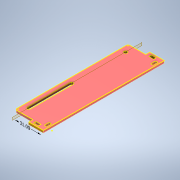
# Autodesk Inventor part: chassis_1_2
Saved by Autodesk Inventor 2022 (Build 260153000, 153)
## iProperties
Created: 2023-03-24
Part Number: chassis_1_2
Material: 一般
Document SubType Name: Modeling
Designer: Johnny Jou
Density: 79.16 g/cm^3
Appearance: 熔接 - 黃銅
Mass: 1010.18 g
Surface Area: 100.717 cm^2
Volume: 12.7613 cm^3
Author: Johnny Jou
Autodesk Inventor part; units mm, degrees
ref_plane "YZ Plane" through (0, 0, 0) normal (1, 0, 0) x (0, 1, 0)
ref_plane "XZ Plane" through (0, 0, 0) normal (0, 1, 0) x (-1, 0, 0)
ref_plane "XY Plane" through (0, 0, 0) normal (0, 0, 1) x (1, 0, 0)
sketch "草圖1" plane through (0, 0, 0) normal (0, 1, 0) x (-1, 0, 0)
  line L0 (0, 0) -> (0, -140)
  line L1 (15, -140) -> (15, 0)
  line L2 (6, 0) -> (6, 3)
  line L3 (6, 3) -> (14.1, 3)
  line L4 (14.1, 3) -> (14.1, 0)
  line L5 (15, 0) -> (14.1, 0)
  line L6 (6, 0) -> (0, 0)
  line L7 (6, -140) -> (6, -143)
  line L8 (6, -143) -> (14.1, -143)
  line L9 (14.1, -143) -> (14.1, -140)
  line L10 (0, -140) -> (6, -140)
  line L11 (14.1, -140) -> (15, -140)
  dimension "d1" = 15
  dimension "d2" = 3
  dimension "d3" = 8.1
  dimension "d4" = 6
  dimension "d5" = 3
  dimension "d6" = 140
  dimension "d7" = 6
  dimension "d8" = 8.1
  dimension "d9" = 15
  dimension "d10" = 140
  constraints: 24 end point, 7 parallel, 4 horizontal, 2 perpendicular, 1 coincident
  measures "d1" distance of L1.end L0.start
  measures "d2" distance of L3.end L4.end
  measures "d3" distance of L2.end L3.end
  measures "d4" distance between parallel lines of L0 L2
  measures "d5" distance of L8.end L9.end
  measures "d6" distance of L0.start L0.end
  measures "d7" distance between parallel lines of L0 L7
  measures "d8" distance of L7.end L8.end
  measures "d9" distance between parallel lines of L0 L1
  measures "d10" distance of L1.start L1.end
extrude "擠出1" add sketch "草圖1" along normal blind 3
sketch "草圖2" plane through (0, 3, 0) normal (0, 1, 0) x (1, 0, 0)
  line L0 (-11, 1) -> (-8, 1)
  line L1 (-8, 1) -> (-8, 7)
  line L2 (-8, 7) -> (-11, 7)
  line L3 (-11, 7) -> (-11, 1)
  line L4 (0, 0) -> (0, 140) projected
  line L5 (-6, 0) -> (0, 0) projected
  line L6 (-11, 133) -> (-8, 133)
  line L7 (-8, 133) -> (-8, 139)
  line L8 (-8, 139) -> (-11, 139)
  line L9 (-11, 139) -> (-11, 133)
  line L10 (0, 140) -> (-6, 140) projected
  line L11 (-15, 140) -> (-15, 0) projected
  dimension "d13" = 6
  dimension "d14" = 3
  dimension "d16" = 1
  dimension "d17" = 6
  dimension "d18" = 3
  dimension "d20" = 1
  dimension "d33" = 4
  dimension "d34" = 4
  constraints: 16 end point, 4 parallel, 2 horizontal, 2 perpendicular
  measures "d13" distance of L2.end L0.start
  measures "d14" distance of L1.end L2.end
  measures "d16" distance between parallel lines of L5 L0
  measures "d17" distance of L8.end L6.start
  measures "d18" distance of L6.start L6.end
  measures "d20" distance between parallel lines of L10 L8
  measures "d33" distance between parallel lines of L11 L3
  measures "d34" distance between parallel lines of L11 L9
extrude "擠出2" cut sketch "草圖2" against normal up to surface (3 mm away)
sketch "草圖4" plane through (0, 3, 0) normal (0, 1, 0) x (1, 0, 0)
  line L0 (-44, 0) -> (-15, 0)
  line L1 (-15, 0) -> (-15, 140)
  line L2 (-15, 140) -> (-44, 140)
  line L3 (-46, 138) -> (-46, 2)
  line L4 (-15, 140) -> (-15, 0) projected
  line L5 (0, 140) -> (-6, 140) projected
  line L6 (-6, 0) -> (0, 0) projected
  line L7 (-39, 10) -> (-39, 63) construction
  line L8 (-37, 10) -> (-37, 63)
  line L9 (-41, 63) -> (-41, 10)
  arc A0 (-41, 10) -> (-37, 10) centre (-39, 10) ccw
  arc A1 (-37, 63) -> (-41, 63) centre (-39, 63) ccw
  circle A2 centre (-39, 130) radius 2
  arc A3 (-46, 2) -> (-44, 0) centre (-44, 2) ccw
  arc A4 (-44, 140) -> (-46, 138) centre (-44, 138) ccw
  point P0 (-39, 36.5)
  dimension "d23" = 31
  dimension "d24" = 4
  dimension "d25" = 53
  dimension "d26" = 5
  dimension "d27" = 10
  dimension "d29" = 2
  dimension "d32" = 10
  constraints: 16 end point, 8 point on circle, 8 tangent, 5 centre point, 3 collinear, 3 parallel, 2 equal radius, 1 horizontal, 1 midpoint, 1 perpendicular, 1 vertical, 1 vertical alignment
  measures "d23" distance between parallel lines of L1 L3
  measures "d24" distance between parallel lines of L8 L9
  measures "d25" distance of L7.end L7.start
  measures "d26" distance between parallel lines of L3 L9
  measures "d27" distance from line of L0 L7.start
  measures "d29" radius of A3
  measures "d32" distance from line of A2.centre L2
extrude "擠出3" add sketch "草圖4" against normal up to surface (3 mm away)
sketch "草圖6" plane through (0, 3, 0) normal (0, 1, 0) x (1, 0, 0)
  circle A0 centre (-39, 130) radius 2 projected
  arc A1 (-41, 10) -> (-37, 10) centre (-39, 10) ccw projected
  line L0 (-41, 10) -> (-41, 63) projected
  arc A2 (-37, 63) -> (-41, 63) centre (-39, 63) ccw projected
  line L1 (-37, 63) -> (-37, 10) projected
  line L2 (-8, 7) -> (-8, 1) projected
  line L3 (-8, 1) -> (-11, 1) projected
  line L4 (-11, 1) -> (-11, 7) projected
  line L5 (-11, 7) -> (-8, 7) projected
  line L6 (-8, 133) -> (-11, 133) projected
  line L7 (-11, 133) -> (-11, 139) projected
  line L8 (-11, 139) -> (-8, 139) projected
  line L9 (-8, 139) -> (-8, 133) projected
  line L10 (0, 0) -> (0, 140) projected
  line L11 (0, 140) -> (-6, 140) projected
  line L12 (-6, 140) -> (-6, 143) projected
  line L13 (-6, 143) -> (-14.1, 143) projected
  line L14 (-14.1, 143) -> (-14.1, 140) projected
  line L15 (-14.1, 140) -> (-44, 140) projected
  arc A3 (-44, 140) -> (-46, 138) centre (-44, 138) ccw projected
  line L16 (-46, 138) -> (-46, 2) projected
  arc A4 (-46, 2) -> (-44, 0) centre (-44, 2) ccw projected
  line L17 (-44, 0) -> (-14.1, 0) projected
  line L18 (-14.1, 0) -> (-14.1, -3) projected
  line L19 (-14.1, -3) -> (-6, -3) projected
  line L20 (-6, -3) -> (-6, 0) projected
  line L21 (-6, 0) -> (0, 0) projected
  line L22 (-6, 140) -> (-6, 143) projected
  line L23 (-6, 0) -> (-6, 140)
  constraints: 2 end point, 1 collinear
extrude "擠出4" cut sketch "草圖6" against normal blind 3 contours L21 L23 L11 L10
ref_plane "工作平面1" through (-39, 3, -10) normal (1, 0, 0) x (0, 0, -1)
sketch "草圖8" plane through (0, 3, 0) normal (0, 1, 0) x (1, 0, 0)
  line L0 (-6, -3) -> (-6, 143) projected
  line L1 (-6, -3) -> (-20.1, -3)
  line L2 (-20.1, -3) -> (-20.1, -5)
  line L3 (-20.1, -5) -> (-6, -5)
  line L4 (-6, -5) -> (-6, -3)
  line L5 (-44, 0) -> (-14.1, 0) projected
  line L6 (-20.1, -5) -> (-24.1, -5)
  line L7 (-24.1, -5) -> (-24.1, 0)
  line L8 (-24.1, 0) -> (-20.1, 0)
  line L9 (-20.1, 0) -> (-20.1, -5)
  line L10 (-14.1, 0) -> (-14.1, -3) projected
  line L11 (-6, 143) -> (-20.1, 143)
  line L12 (-20.1, 143) -> (-20.1, 145)
  line L13 (-20.1, 145) -> (-6, 145)
  line L14 (-6, 145) -> (-6, 143)
  line L15 (-14.1, 140) -> (-44, 140) projected
  line L16 (-20.1, 145) -> (-24.1, 145)
  line L17 (-24.1, 145) -> (-24.1, 140)
  line L18 (-24.1, 140) -> (-20.1, 140)
  line L19 (-20.1, 140) -> (-20.1, 145)
  line L20 (-14.1, 143) -> (-14.1, 140) projected
  point P0 (0, 0)
  dimension "d40" = 6
  dimension "d41" = 2
  dimension "d42" = 4
  dimension "d45" = 6
  dimension "d46" = 2
  dimension "d47" = 4
  constraints: 32 end point, 8 parallel, 4 horizontal, 4 perpendicular, 2 point on line
  measures "d40" distance between parallel lines of L10 L9
  measures "d41" distance between parallel lines of L1 L3
  measures "d42" distance between parallel lines of L2 L7
  measures "d45" distance between parallel lines of L20 L19
  measures "d46" distance of L11.end L12.end
  measures "d47" distance between parallel lines of L19 L17
extrude "擠出5" add sketch "草圖8" against normal up to surface (3 mm away) contours L11 L12 L13 L14 | L4 L3 L2 L1 | L2 L6 L7 L5 L9 | L19 L15 L17 L16 L12
sketch "草圖9" plane through (0, 3, 0) normal (0, 1, 0) x (1, 0, 0)
  line L0 (-6, -5) -> (-6, 145) projected
  line L1 (-6, 145) -> (-24.1, 145) projected
  line L2 (-24.1, 145) -> (-24.1, 140) projected
  line L3 (-24.1, 140) -> (-44, 140) projected
  arc A0 (-44, 140) -> (-46, 138) centre (-44, 138) ccw projected
  line L4 (-46, 138) -> (-46, 2) projected
  arc A1 (-46, 2) -> (-44, 0) centre (-44, 2) ccw projected
  line L5 (-44, 0) -> (-24.1, 0) projected
  line L6 (-24.1, 0) -> (-24.1, -5) projected
  line L7 (-24.1, -5) -> (-6, -5) projected
  line L8 (-14.1, -3) -> (-20.1, -3) projected
  line L9 (-20.1, -3) -> (-20.1, 0) projected
  line L10 (-20.1, 0) -> (-14.1, 0) projected
  line L11 (-14.1, 0) -> (-14.1, -3) projected
  line L12 (-20.1, 140) -> (-20.1, 143) projected
  line L13 (-20.1, 143) -> (-14.1, 143) projected
  line L14 (-14.1, 143) -> (-14.1, 140) projected
  line L15 (-14.1, 140) -> (-20.1, 140) projected
  circle A2 centre (-39, 130) radius 2 projected
  arc A3 (-41, 10) -> (-37, 10) centre (-39, 10) ccw projected
  line L16 (-41, 10) -> (-41, 63) projected
  arc A4 (-37, 63) -> (-41, 63) centre (-39, 63) ccw projected
  line L17 (-37, 63) -> (-37, 10) projected
  line L18 (-8, 7) -> (-8, 1) projected
  line L19 (-8, 1) -> (-11, 1) projected
  line L20 (-11, 1) -> (-11, 7) projected
  line L21 (-11, 7) -> (-8, 7) projected
  line L22 (-8, 133) -> (-11, 133) projected
  line L23 (-11, 133) -> (-11, 139) projected
  line L24 (-11, 139) -> (-8, 139) projected
  line L25 (-8, 139) -> (-8, 133) projected
  point P0 (0, 0)
equation "\"d10\" = d6"
equation "\"d20\" = d16"
